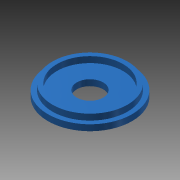
# Autodesk Inventor part: HubCover
Saved by Autodesk Inventor 2014 SP1 (Build 180222100, 222)
## iProperties
Created: 2017-01-04
Part Number: HubCover
Material: Generic
Document SubType Name: Modeling
Designer: danielsikar
Density: 1 g/cm^3
Appearance: Cyan
Author: danielsikar
Autodesk Inventor part; units mm, degrees
ref_plane "YZ Plane" through (0, 0, 0) normal (1, 0, 0) x (0, 1, 0)
ref_plane "XZ Plane" through (0, 0, 0) normal (0, 1, 0) x (-1, 0, 0)
ref_plane "XY Plane" through (0, 0, 0) normal (0, 0, 1) x (1, 0, 0)
sketch "Sketch1" plane through (0, 0, 0) normal (0, 0, 1) x (1, 0, 0)
  circle A0 centre (0, 0) radius 7
  dimension "d0" = 14
  constraints: 1 centre point, 1 coincident
  measures "d0" diameter of A0
extrude "Extrusion1" add sketch "Sketch1" along normal blind 1
sketch "Sketch2" plane through (0, 0, 1) normal (0, 0, 1) x (1, 0, 0)
  circle A0 centre (0, 0) radius 7 projected
  circle A1 centre (0, 0) radius 2.2
  dimension "d3" = 4.4
  constraints: 1 centre point, 1 coincident
  measures "d3" diameter of A1
extrude "Extrusion2" cut sketch "Sketch2" against normal blind 1 contours A1
sketch "Sketch3" plane through (0, 0, 1) normal (0, 0, 1) x (1, 0, 0)
  circle A0 centre (0, 0) radius 7 projected
  circle A1 centre (0, 0) radius 6.25
  circle A2 centre (0, 0) radius 5.5
  dimension "d6" = 12.5
  dimension "d7" = 11
  constraints: 2 centre point, 2 coincident
  measures "d6" diameter of A1
  measures "d7" diameter of A2
extrude "Extrusion3" add sketch "Sketch3" along normal blind 1 contours A1
body "Solid1"
